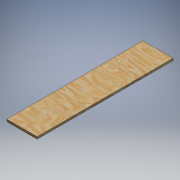
# Autodesk Inventor part: Base_wood
Saved by Autodesk Inventor 2016 SP2 (Build 200236200, 236)
## iProperties
Created: 2017-08-26
Part Number: Base_wood
Material: Generic
Document SubType Name: Modeling
Designer: Admin
Density: 1 g/cm^3
Appearance: Default
Author: Admin
Autodesk Inventor part; units mm, degrees
ref_plane "YZ Plane" through (0, 0, 0) normal (1, 0, 0) x (0, 1, 0)
ref_plane "XZ Plane" through (0, 0, 0) normal (0, 1, 0) x (-1, 0, 0)
ref_plane "XY Plane" through (0, 0, 0) normal (0, 0, 1) x (1, 0, 0)
sketch "Sketch1" plane through (0, 0, 0) normal (0, 0, 1) x (1, 0, 0)
  line L0 (-100, 450) -> (100, 450)
  line L1 (100, 450) -> (100, -450)
  line L2 (100, -450) -> (-100, -450)
  line L3 (-100, -450) -> (-100, 450)
  line L4 (-100, 450) -> (100, -450) construction
  point P0 (0, 0)
  point P1 (0, 0)
  dimension "d0" = 900
  dimension "d1" = 200
  constraints: 10 end point, 2 parallel, 1 coincident, 1 horizontal, 1 midpoint, 1 perpendicular
  measures "d0" distance of L2.end L0.start
  measures "d1" distance of L0.start L0.end
extrude "Extrusion1" add sketch "Sketch1" along normal blind 15
body "Solid1"
